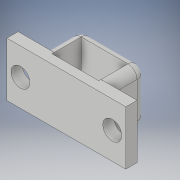
# Autodesk Inventor part: USBholder version 1
Saved by Autodesk Inventor 2019 (Build 230136000, 136)
## iProperties
Created: 2019-01-16
Part Number: USBholder version 1
Material: Generic
Document SubType Name: Modeling
Designer: ashle
Density: 1 g/cm^3
Appearance: Default
Author: ashle
Autodesk Inventor part; units mm, degrees
ref_plane "YZ Plane" through (0, 0, 0) normal (1, 0, 0) x (0, 1, 0)
ref_plane "XZ Plane" through (0, 0, 0) normal (0, 1, 0) x (-1, 0, 0)
ref_plane "XY Plane" through (0, 0, 0) normal (0, 0, 1) x (1, 0, 0)
sketch "Sketch1" plane through (0, 0, 0) normal (0, 1, 0) x (-1, 0, 0)
  line L0 (5.2, 3.25) -> (-5.2, 3.25)
  line L1 (-5.2, 3.25) -> (-5.2, -3.25)
  line L2 (-5.2, -3.25) -> (5.2, -3.25)
  line L3 (5.2, -3.25) -> (5.2, 3.25)
  line L4 (0, -3.25) -> (0, 3.25) construction
  line L5 (5.2, 0) -> (-5.2, 0) construction
  line L6 (7.2, -5.25) -> (-7.2, -5.25)
  line L7 (-7.2, -5.25) -> (-7.2, 5.25)
  line L8 (-7.2, 5.25) -> (7.2, 5.25)
  line L9 (7.2, 5.25) -> (7.2, -5.25)
  line L10 (-13.2, 2.75) -> (-7.2, 2.75)
  line L11 (-7.2, 2.75) -> (-7.2, 5.25)
  line L12 (-7.2, 5.25) -> (-13.2, 5.25)
  line L13 (-13.2, 5.25) -> (-13.2, 2.75)
  line L14 (7.2, 2.75) -> (13.2, 2.75)
  line L15 (13.2, 2.75) -> (13.2, 5.25)
  line L16 (13.2, 5.25) -> (7.2, 5.25)
  line L17 (7.2, 5.25) -> (7.2, 2.75)
  point P0 (0, 0)
  dimension "d0" = 10.4
  dimension "d1" = 6.5
  dimension "d4" = 2
  dimension "d5" = 2
  dimension "d6" = 2
  dimension "d7" = 2
  dimension "d8" = 2.5
  dimension "d9" = 2.5
  dimension "d10" = 6
  dimension "d11" = 6
  constraints: 36 end point, 8 parallel, 6 midpoint, 4 collinear, 4 horizontal, 4 perpendicular
  measures "d0" distance between parallel lines of L1 L3
  measures "d1" distance between parallel lines of L2 L0
  measures "d4" distance between parallel lines of L8 L0
  measures "d5" distance between parallel lines of L2 L6
  measures "d6" distance between parallel lines of L7 L1
  measures "d7" distance between parallel lines of L9 L3
  measures "d8" distance between parallel lines of L16 L14
  measures "d9" distance between parallel lines of L10 L12
  measures "d10" distance between parallel lines of L15 L9
  measures "d11" distance between parallel lines of L13 L7
extrude "Extrusion2" add sketch "Sketch1" along normal blind 12
sketch "Sketch2" plane through (13.2, 0, 2.75) normal (0, 0, -1) x (-1, 0, 0)
  line L0 (26.4, 0) -> (20.4, 0) construction
  line L1 (20.4, 0) -> (20.4, 12) construction
  line L2 (20.4, 12) -> (26.4, 12) construction
  line L3 (26.4, 12) -> (26.4, 0) construction
  line L4 (20.4, 0) -> (26.4, 0) construction
  line L5 (26.4, 0) -> (26.4, 12) construction
  line L6 (20.4, 0) -> (20.4, 12) construction
  line L7 (20.4, 12) -> (26.4, 12) construction
  line L8 (23.4, 0) -> (23.4, 12) construction
  line L9 (26.4, 6) -> (20.4, 6) construction
  circle A0 centre (15.4635, 5.7038) radius 3.0285
  circle A1 centre (23.4, 6) radius 2.1
  line L10 (13.2, -1.4538) -> (13.2, 18.2002) construction
  circle A2 centre (3, 6) radius 2.1
  point P0 (13.2, 0)
  point P1 (23.4, 6)
  dimension "d15" = 4.2
  constraints: 14 end point, 5 midpoint, 4 collinear, 3 centre point, 2 parallel, 1 coincident, 1 horizontal, 1 perpendicular, 1 symmetric about line, 1 vertical, 1 other
  measures "d15" diameter of A1
extrude "Extrusion3" cut sketch "Sketch2" against normal up to surface (2.5 mm away) contours A1 | A2
fillet "Fillet1" radius 2 4 edges at (7.2, 6, -5.25) (-7.2, 6, -5.25) (0, 12, -5.25) (0, 0, -5.25)
fillet "Fillet2" radius 2 8 edges at (-6.6142, 11.4142, -4.6642) (-7.2, 12, -0.25) (6.6142, 11.4142, -4.6642) (7.2, 12, -0.2501) (6.6142, 0.5858, -4.6642) (7.2, 0, -0.2501) (-6.6142, 0.5858, -4.6642) (-7.2, 0, -0.25)
equation "\"d5\" = d4"
equation "\"d6\" = d4"
equation "\"d7\" = d4"
equation "\"d9\" = d8"
equation "\"d10\" = d11"
body "Solid2"
